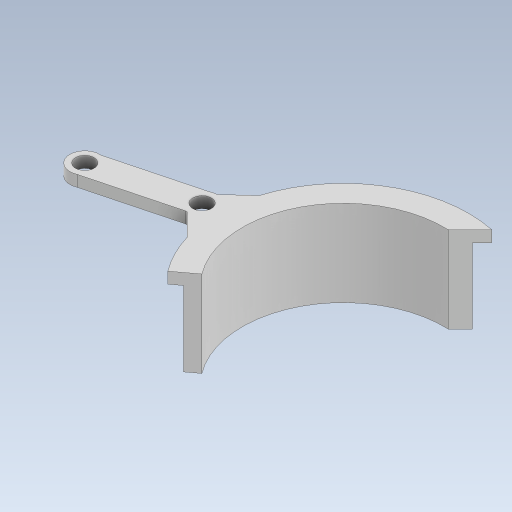
# Autodesk Inventor part: Right Hand
Saved by Autodesk Inventor 2023.5 (Build 275446000, 446)
## iProperties
Created: 2025-10-05
Part Number: Right Hand
Material: Generic
Document SubType Name: Modeling
Designer: Guntur
Density: 1 g/cm^3
Appearance: Default
Author: Guntur
## iProperties of the stored document Right Hand_3DPrint.ipt
Created: 2025-10-05
Part Number: Right Hand_3DPrint
Material: Generic
Document SubType Name: Modeling
Designer: Guntur
Density: 1 g/cm^3
Appearance: Default
Author: Guntur
Autodesk Inventor part; units mm, degrees
ref_plane "YZ Plane" through (0, 0, 0) normal (1, 0, 0) x (0, 1, 0)
ref_plane "XZ Plane" through (0, 0, 0) normal (0, 1, 0) x (-1, 0, 0)
ref_plane "XY Plane" through (0, 0, 0) normal (0, 0, 1) x (1, 0, 0)
sketch "Sketch1" plane through (0, 0, 0) normal (0, 1, 0) x (-1, 0, 0)
  arc A0 (-46.1959, -183.8031) -> (0.2724, -149.0945) centre (-22.9311, -166.4898) ccw
  arc A1 (-47.3976, -184.7007) -> (1.4742, -148.1969) centre (-22.9311, -166.4898) ccw
  arc A2 (-49.8012, -186.496) -> (3.8777, -146.4016) centre (-22.9311, -166.4898) ccw
  circle A3 centre (15.0259, -166.701) radius 2.5
  circle A4 centre (15.0259, -166.701) radius 4
  line L0 (42.3478, -163.6082) -> (16.693, -170.3371)
  circle A5 centre (40.0259, -160.351) radius 2.5
  circle A6 centre (40.0259, -160.351) radius 4
  line L1 (12.7041, -163.4439) -> (38.3588, -156.715)
  line L2 (-22.9311, -166.4898) -> (9.5689, -166.4898) construction
  line L3 (15.0259, -162.701) -> (9.1421, -156.8172)
  line L4 (15.0259, -162.701) -> (23.347, -162.701) construction
  line L5 (40.0259, -160.351) -> (40.0259, -166.701)
  line L6 (15.0259, -166.701) -> (40.0259, -160.351)
  line L7 (3.8777, -146.4016) -> (-49.8012, -186.496)
  line L8 (-34.5984, -197.8924) -> (-31.5136, -194.1907)
  line L9 (15.0259, -170.701) -> (21.3292, -170.701) construction
  line L10 (15.0259, -170.701) -> (9.1421, -176.1623)
  circle A7 centre (-22.9311, -166.4898) radius 27
  line L11 (-49.8012, -186.496) -> (-49.8012, -206)
  line L12 (-49.8012, -206) -> (-29.8012, -206)
  line L13 (-29.8012, -206) -> (-29.8012, -199.2777)
  line L14 (-29.8012, -199.2777) -> (-24.7141, -194.1907)
  line L15 (-29.8012, -199.2777) -> (-22.607, -199.2777) construction
  line L16 (-24.7141, -194.1907) -> (-23.9923, -193.4689)
  line L17 (-31.5136, -194.1907) -> (-30.1178, -192.5157)
  point P0 (0, -166)
  point P1 (10.3976, -163.1063)
  point P2 (10.5689, -166.4898)
  point P3 (-56.4309, -166.6014)
  point P4 (11.7433, -168.9867)
  point P5 (15.4503, -162.7236)
  point P6 (39.6016, -164.3285)
  point P7 (-46.6192, -190.1778)
  point P8 (0.7569, -142.8017)
  point P9 (19.0611, -162.9823)
  point P10 (1.0736, -148.4961)
  point P11 (-46.9971, -184.4015)
  point P12 (0.2724, -149.0945)
  point P13 (-32.5494, -195.4335)
  point P14 (-27.2114, -196.6879)
  point P15 (-1.3299, -150.2913)
  dimension "d18" = 67
  dimension "d14" = 135
  dimension "d17" = 25
  dimension "d19" = 61
  dimension "d20" = 58
  dimension "d21" = 8
  dimension "d22" = 5
  dimension "d23" = 8
  dimension "d24" = 5
  dimension "d25" = 19
  dimension "d27" = 54
  dimension "d28" = 20
  dimension "d29" = 45
  constraints: 36 end point, 14 point on circle, 7 centre point, 6 coincident, 6 point on line, 4 horizontal, 2 equal length, 2 perpendicular, 2 vertical, 13 other
  measures "d14" angle of L4 L3
  measures "d17" horizontal distance of point (15.026, -166.701) A6.centre
  measures "d19" diameter of A1
  measures "d20" diameter of A0
  measures "d21" diameter of A4
  measures "d22" diameter of A3
  measures "d23" diameter of A6
  measures "d24" diameter of A5
  measures "d25" distance of L7.end L8.start
  measures "d27" diameter of A7
  measures "d28" distance of L11.end L12.end
  measures "d29" angle of L15 L14
extrude "Extrusion1" add sketch "Sketch1" along normal blind 3 contours A1 L7 A2 L14 | A2 L3 A4 L10 | A4 L1 | A4 L1 | A4 L6 A6 L0 | L1 A6 L6 A4 | A6 L6 A5 L5 L0 | L0 L5 A6 | A6 L0 L5 A5 L6 | L0 A6 L5
extrude "Extrusion2" add sketch "Sketch1" along normal blind 3 and the other way blind 20 contours L14 L16 A7 L7 A0 | A0 L7 A1 L14
body "Solid1"
